Autodesk Inventor part; units mm, degrees
(part 2 of 2)
  spline S278 degree 2 poles (87.85, 28.3635) (87.85, 28.6167) (87.7568, 28.9368) (87.6738, 29.0239) knots 0 0 0 1 2 2 2
  spline S279 degree 2 poles (87.6738, 29.0239) (87.6008, 29.1049) (87.4489, 29.1657) (87.3597, 29.1657) knots 0 0 0 1 2 2 2
  spline S280 degree 2 poles (87.3597, 29.1657) (87.1531, 29.1657) (86.908, 28.8699) (86.908, 28.5904) knots 0 0 0 1 2 2 2
  spline S281 degree 2 poles (86.908, 28.5904) (86.908, 28.4323) (86.989, 28.2277) (87.0781, 28.1548) knots 0 0 0 1 2 2 2
  spline S282 degree 2 poles (87.0781, 28.1548) (87.143, 28.1021) (87.303, 28.0677) (87.3962, 28.0677) knots 0 0 0 1 2 2 2
  spline S283 degree 2 poles (87.3962, 28.0677) (87.5036, 28.0677) (87.7508, 28.1426) (87.8439, 28.2054) knots 0 0 0 1 2 2 2
  spline S284 degree 2 poles (87.8439, 28.2054) (87.846, 28.2297) (87.85, 28.3128) (87.85, 28.3635) knots 0 0 0 1 2 2 2
  line L255 (90.0826, 29.0138) -> (89.0008, 26.8886)
  line L256 (89.0008, 26.8886) -> (88.6442, 26.8886)
  line L257 (88.6442, 26.8886) -> (89.7868, 29.0948)
  line L258 (89.7868, 29.0948) -> (88.4963, 29.0948)
  line L259 (88.4963, 29.0948) -> (88.4963, 29.3886)
  line L260 (88.4963, 29.3886) -> (90.0826, 29.3886)
  line L261 (90.0826, 29.3886) -> (90.0826, 29.0138)
  line L262 (93.2613, 29.3886) -> (92.6332, 26.8886)
  line L263 (92.6332, 26.8886) -> (92.2605, 26.8886)
  line L264 (92.2605, 26.8886) -> (91.752, 28.9631)
  line L265 (91.752, 28.9631) -> (91.2576, 26.8886)
  line L266 (91.2576, 26.8886) -> (90.8889, 26.8886)
  line L267 (90.8889, 26.8886) -> (90.2508, 29.3886)
  line L268 (90.2508, 29.3886) -> (90.5931, 29.3886)
  line L269 (90.5931, 29.3886) -> (91.0956, 27.316)
  line L270 (91.0956, 27.316) -> (91.5939, 29.3886)
  line L271 (91.5939, 29.3886) -> (91.9323, 29.3886)
  line L272 (91.9323, 29.3886) -> (92.4347, 27.2917)
  line L273 (92.4347, 27.2917) -> (92.9351, 29.3886)
  line L274 (92.9351, 29.3886) -> (93.2613, 29.3886)
  line L275 (95.0076, 26.8886) -> (94.6916, 26.8886)
  line L276 (94.6916, 26.8886) -> (94.6916, 27.9583)
  spline S285 degree 2 poles (94.6916, 27.9583) (94.6916, 28.0879) (94.6673, 28.3108) (94.6308, 28.3776) knots 0 0 0 1 2 2 2
  spline S286 degree 2 poles (94.6308, 28.3776) (94.5923, 28.4485) (94.4546, 28.5174) (94.3371, 28.5174) knots 0 0 0 1 2 2 2
  spline S287 degree 2 poles (94.3371, 28.5174) (94.2196, 28.5174) (93.9704, 28.3918) (93.8508, 28.2905) knots 0 0 0 1 2 2 2
  line L277 (93.8508, 28.2905) -> (93.8508, 26.8886)
  line L278 (93.8508, 26.8886) -> (93.5348, 26.8886)
  line L279 (93.5348, 26.8886) -> (93.5348, 29.5)
  line L280 (93.5348, 29.5) -> (93.8508, 29.5)
  line L281 (93.8508, 29.5) -> (93.8508, 28.5559)
  spline S288 degree 2 poles (93.8508, 28.5559) (93.9926, 28.6835) (94.2661, 28.8173) (94.4201, 28.8173) knots 0 0 0 1 2 2 2
  spline S289 degree 2 poles (94.4201, 28.8173) (94.6956, 28.8173) (95.0076, 28.4526) (95.0076, 28.1062) knots 0 0 0 1 2 2 2
  line L282 (95.0076, 28.1062) -> (95.0076, 26.8886)
  line L283 (98.0202, 26.8886) -> (96.4785, 26.8886)
  line L284 (96.4785, 26.8886) -> (96.4785, 27.2431)
  spline S290 degree 2 poles (96.4785, 27.2431) (96.6446, 27.3991) (96.9404, 27.6888) (97.0822, 27.8448) knots 0 0 0 1 2 2 2
  spline S291 degree 2 poles (97.0822, 27.8448) (97.3679, 28.1588) (97.5765, 28.5357) (97.5765, 28.7362) knots 0 0 0 1 2 2 2
  spline S292 degree 2 poles (97.5765, 28.7362) (97.5765, 28.8416) (97.5117, 28.9996) (97.4529, 29.0502) knots 0 0 0 1 2 2 2
  spline S293 degree 2 poles (97.4529, 29.0502) (97.3942, 29.1009) (97.2402, 29.1515) (97.147, 29.1515) knots 0 0 0 1 2 2 2
  spline S294 degree 2 poles (97.147, 29.1515) (97.0579, 29.1515) (96.8755, 29.107) (96.7925, 29.0725) knots 0 0 0 1 2 2 2
  spline S295 degree 2 poles (96.7925, 29.0725) (96.7216, 29.0442) (96.5899, 28.9631) (96.5494, 28.9348) knots 0 0 0 1 2 2 2
  line L285 (96.5494, 28.9348) -> (96.5311, 28.9348)
  line L286 (96.5311, 28.9348) -> (96.5311, 29.2913)
  spline S296 degree 2 poles (96.5311, 29.2913) (96.6345, 29.342) (97.0052, 29.4412) (97.1713, 29.4412) knots 0 0 0 1 2 2 2
  spline S297 degree 2 poles (97.1713, 29.4412) (97.5218, 29.4412) (97.9169, 29.0705) (97.9169, 28.7545) knots 0 0 0 1 2 2 2
  spline S298 degree 2 poles (97.9169, 28.7545) (97.9169, 28.6066) (97.848, 28.3594) (97.7872, 28.2541) knots 0 0 0 1 2 2 2
  spline S299 degree 2 poles (97.7872, 28.2541) (97.7264, 28.1447) (97.5502, 27.9299) (97.4529, 27.8266) knots 0 0 0 1 2 2 2
  spline S300 degree 2 poles (97.4529, 27.8266) (97.2949, 27.6544) (96.908, 27.2857) (96.7925, 27.1783) knots 0 0 0 1 2 2 2
  line L287 (96.7925, 27.1783) -> (98.0202, 27.1783)
  line L288 (98.0202, 27.1783) -> (98.0202, 26.8886)
  spline S301 degree 2 poles (99.8699, 27.6827) (99.8699, 27.5024) (99.7544, 27.1945) (99.649, 27.081) knots 0 0 0 1 2 2 2
  spline S302 degree 2 poles (99.649, 27.081) (99.5437, 26.9676) (99.2297, 26.8359) (99.0352, 26.8359) knots 0 0 0 1 2 2 2
  spline S303 degree 2 poles (99.0352, 26.8359) (98.8569, 26.8359) (98.5084, 26.9149) (98.3808, 26.9777) knots 0 0 0 1 2 2 2
  line L289 (98.3808, 26.9777) -> (98.3808, 27.3323)
  line L290 (98.3808, 27.3323) -> (98.4051, 27.3323)
  spline S304 degree 2 poles (98.4051, 27.3323) (98.4436, 27.3039) (98.5875, 27.231) (98.6746, 27.1985) knots 0 0 0 1 2 2 2
  spline S305 degree 2 poles (98.6746, 27.1985) (98.7738, 27.1641) (98.9379, 27.1256) (99.0413, 27.1256) knots 0 0 0 1 2 2 2
  spline S306 degree 2 poles (99.0413, 27.1256) (99.1426, 27.1256) (99.333, 27.1985) (99.4019, 27.2776) knots 0 0 0 1 2 2 2
  spline S307 degree 2 poles (99.4019, 27.2776) (99.4647, 27.3525) (99.5295, 27.5511) (99.5295, 27.6848) knots 0 0 0 1 2 2 2
  spline S308 degree 2 poles (99.5295, 27.6848) (99.5295, 27.8185) (99.4566, 27.9887) (99.3877, 28.0454) knots 0 0 0 1 2 2 2
  spline S309 degree 2 poles (99.3877, 28.0454) (99.3168, 28.1082) (99.1061, 28.1609) (98.9785, 28.1609) knots 0 0 0 1 2 2 2
  spline S310 degree 2 poles (98.9785, 28.1609) (98.8407, 28.1609) (98.5672, 28.1183) (98.4841, 28.1001) knots 0 0 0 1 2 2 2
  line L291 (98.4841, 28.1001) -> (98.4841, 29.3886)
  line L292 (98.4841, 29.3886) -> (99.8557, 29.3886)
  line L293 (99.8557, 29.3886) -> (99.8557, 29.0948)
  line L294 (99.8557, 29.0948) -> (98.8063, 29.0948)
  line L295 (98.8063, 29.0948) -> (98.8063, 28.4283)
  spline S311 degree 2 poles (98.8063, 28.4283) (98.867, 28.4364) (98.9845, 28.4425) (99.0332, 28.4425) knots 0 0 0 1 2 2 2
  spline S312 degree 2 poles (99.0332, 28.4425) (99.2256, 28.4425) (99.491, 28.3797) (99.6126, 28.2865) knots 0 0 0 1 2 2 2
  spline S313 degree 2 poles (99.6126, 28.2865) (99.7362, 28.1933) (99.8699, 27.9096) (99.8699, 27.6827) knots 0 0 0 1 2 2 2
  spline S314 degree 2 poles (101.2779, 26.844) (101.0348, 26.844) (100.6235, 27.0081) (100.4736, 27.1722) knots 0 0 0 1 2 2 2
  spline S315 degree 2 poles (100.4736, 27.1722) (100.3237, 27.3343) (100.1596, 27.8205) (100.1596, 28.1365) knots 0 0 0 1 2 2 2
  spline S316 degree 2 poles (100.1596, 28.1365) (100.1596, 28.4506) (100.3196, 28.9165) (100.4716, 29.0887) knots 0 0 0 1 2 2 2
  spline S317 degree 2 poles (100.4716, 29.0887) (100.6215, 29.2569) (101.0307, 29.4331) (101.284, 29.4331) knots 0 0 0 1 2 2 2
  spline S318 degree 2 poles (101.284, 29.4331) (101.4096, 29.4331) (101.6304, 29.3967) (101.7236, 29.3683) knots 0 0 0 1 2 2 2
  spline S319 degree 2 poles (101.7236, 29.3683) (101.8046, 29.342) (101.9728, 29.267) (102.0559, 29.2224) knots 0 0 0 1 2 2 2
  line L296 (102.0559, 29.2224) -> (102.0559, 28.8213)
  line L297 (102.0559, 28.8213) -> (102.0295, 28.8213)
  spline S320 degree 2 poles (102.0295, 28.8213) (101.9849, 28.8618) (101.8472, 28.9753) (101.7479, 29.03) knots 0 0 0 1 2 2 2
  spline S321 degree 2 poles (101.7479, 29.03) (101.6527, 29.0827) (101.4278, 29.1495) (101.282, 29.1495) knots 0 0 0 1 2 2 2
  spline S322 degree 2 poles (101.282, 29.1495) (101.1219, 29.1495) (100.8362, 29.0178) (100.7289, 28.8922) knots 0 0 0 1 2 2 2
  spline S323 degree 2 poles (100.7289, 28.8922) (100.6235, 28.7646) (100.506, 28.3776) (100.506, 28.1365) knots 0 0 0 1 2 2 2
  spline S324 degree 2 poles (100.506, 28.1365) (100.506, 27.8793) (100.6296, 27.5085) (100.737, 27.3809) knots 0 0 0 1 2 2 2
  spline S325 degree 2 poles (100.737, 27.3809) (100.8423, 27.2573) (101.1239, 27.1317) (101.282, 27.1317) knots 0 0 0 1 2 2 2
  spline S326 degree 2 poles (101.282, 27.1317) (101.4258, 27.1317) (101.6709, 27.2026) (101.7661, 27.2553) knots 0 0 0 1 2 2 2
  spline S327 degree 2 poles (101.7661, 27.2553) (101.8573, 27.3079) (101.9931, 27.4173) (102.0315, 27.4558) knots 0 0 0 1 2 2 2
  line L298 (102.0315, 27.4558) -> (102.0559, 27.4558)
  line L299 (102.0559, 27.4558) -> (102.0559, 27.0588)
  spline S328 degree 2 poles (102.0559, 27.0588) (101.9728, 27.0203) (101.8269, 26.9494) (101.7236, 26.9169) knots 0 0 0 1 2 2 2
  spline S329 degree 2 poles (101.7236, 26.9169) (101.6142, 26.8805) (101.4278, 26.844) (101.2779, 26.844) knots 0 0 0 1 2 2 2
  point P0 (-1.739, -2.5)
  dimension "d13" = 6
  dimension "d14" = 3
  constraints: 6 other
  measures "d13" distance from line of L0.end L4
  measures "d14" distance from line of L9 L0.end
extrude "Extrusion3" add sketch "Skizze3" along normal blind 0.01
